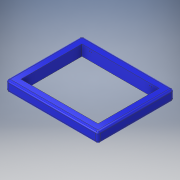
# Autodesk Inventor part: Wrap-Around Bumpers
Saved by Autodesk Inventor 2019 (Build 230136000, 136)
## iProperties
Created: 2018-11-17
Part Number: Wrap-Around Bumpers
Material: Generic
Document SubType Name: Modeling
Designer: maste
Density: 1 g/cm^3
Appearance: Default
Author: maste
Autodesk Inventor part; units mm, degrees
ref_plane "YZ Plane" through (0, 0, 0) normal (1, 0, 0) x (0, 1, 0)
ref_plane "XZ Plane" through (0, 0, 0) normal (0, 1, 0) x (-1, 0, 0)
ref_plane "XY Plane" through (0, 0, 0) normal (0, 0, 1) x (1, 0, 0)
sketch "Sketch1" plane through (0, 0, 0) normal (0, 0, 1) x (1, 0, 0)
  line L0 (0, 0) -> (914.4, 0)
  line L1 (914.4, 0) -> (914.4, 723.9)
  line L2 (914.4, 723.9) -> (0, 723.9)
  line L3 (0, 723.9) -> (0, 0)
  line L4 (-88.9, 812.8) -> (1003.3, 812.8)
  line L5 (1003.3, 812.8) -> (1003.3, -88.9)
  line L6 (1003.3, -88.9) -> (-88.9, -88.9)
  line L7 (-88.9, -88.9) -> (-88.9, 812.8)
  dimension "d0" = 914.4
  dimension "d1" = 723.9
  dimension "d2" = 88.9
  constraints: 16 end point, 4 parallel, 2 perpendicular, 1 horizontal, 3 other
  measures "d0" distance of L2.end L1.end
  measures "d1" distance of L1.end L0.end
  measures "d2" distance between parallel lines of L2 L4
extrude "Extrusion1" add sketch "Sketch1" along normal blind 127
sketch "Sketch2" plane through (1003.3, -88.9, 0) normal (1, 0, 0) x (0, 0, -1)
  line L0 (-101.3437, 557.5546) -> (-13.411, 557.5546) construction
  line L1 (-13.411, 557.5546) -> (-13.411, 343.9106) construction
  line L2 (-13.411, 343.9106) -> (-101.3437, 343.9106) construction
  line L3 (-101.3437, 343.9106) -> (-101.3437, 557.5546) construction
  line L4 (-99.1602, 555.4971) -> (-99.5233, 555.4971)
  line L5 (-99.5233, 555.4971) -> (-99.5233, 554.4498)
  line L6 (-99.5233, 554.4498) -> (-99.9161, 554.4498)
  line L7 (-99.9161, 554.4498) -> (-99.9161, 555.4971)
  line L8 (-99.9161, 555.4971) -> (-101.2622, 555.4971)
  line L9 (-101.2622, 555.4971) -> (-101.2622, 555.9269)
  line L10 (-101.2622, 555.9269) -> (-99.8988, 557.4978)
  line L11 (-99.8988, 557.4978) -> (-99.5233, 557.4978)
  line L12 (-99.5233, 557.4978) -> (-99.5233, 555.8256)
  line L13 (-99.5233, 555.8256) -> (-99.1602, 555.8256)
  line L14 (-99.1602, 555.8256) -> (-99.1602, 555.4971)
  line L15 (-99.9161, 555.8256) -> (-99.9161, 557.0161)
  line L16 (-99.9161, 557.0161) -> (-100.9411, 555.8256)
  line L17 (-100.9411, 555.8256) -> (-99.9161, 555.8256)
  line L18 (-96.873, 555.4971) -> (-97.2361, 555.4971)
  line L19 (-97.2361, 555.4971) -> (-97.2361, 554.4498)
  line L20 (-97.2361, 554.4498) -> (-97.6288, 554.4498)
  line L21 (-97.6288, 554.4498) -> (-97.6288, 555.4971)
  line L22 (-97.6288, 555.4971) -> (-98.975, 555.4971)
  line L23 (-98.975, 555.4971) -> (-98.975, 555.9269)
  line L24 (-98.975, 555.9269) -> (-97.6115, 557.4978)
  line L25 (-97.6115, 557.4978) -> (-97.2361, 557.4978)
  line L26 (-97.2361, 557.4978) -> (-97.2361, 555.8256)
  line L27 (-97.2361, 555.8256) -> (-96.873, 555.8256)
  line L28 (-96.873, 555.8256) -> (-96.873, 555.4971)
  line L29 (-97.6288, 555.8256) -> (-97.6288, 557.0161)
  line L30 (-97.6288, 557.0161) -> (-98.6539, 555.8256)
  line L31 (-98.6539, 555.8256) -> (-97.6288, 555.8256)
  spline S0 degree 2 poles (-94.6203, 555.4378) (-94.6203, 555.2032) (-94.776, 554.8055) (-94.9069, 554.6721) knots 0 0 0 1 2 2 2
  spline S1 degree 2 poles (-94.9069, 554.6721) (-95.0427, 554.5313) (-95.3836, 554.3856) (-95.5886, 554.3856) knots 0 0 0 1 2 2 2
  spline S2 degree 2 poles (-95.5886, 554.3856) (-95.7936, 554.3856) (-96.132, 554.5239) (-96.2604, 554.6622) knots 0 0 0 1 2 2 2
  spline S3 degree 2 poles (-96.2604, 554.6622) (-96.4185, 554.8277) (-96.5964, 555.3835) (-96.5964, 555.7885) knots 0 0 0 1 2 2 2
  spline S4 degree 2 poles (-96.5964, 555.7885) (-96.5964, 556.1862) (-96.4333, 556.826) (-96.2629, 557.0631) knots 0 0 0 1 2 2 2
  spline S5 degree 2 poles (-96.2629, 557.0631) (-96.0974, 557.2953) (-95.5738, 557.5546) (-95.2304, 557.5546) knots 0 0 0 1 2 2 2
  spline S6 degree 2 poles (-95.2304, 557.5546) (-95.1292, 557.5546) (-94.9513, 557.5348) (-94.8846, 557.5126) knots 0 0 0 1 2 2 2
  line L32 (-94.8846, 557.5126) -> (-94.8846, 557.1199)
  line L33 (-94.8846, 557.1199) -> (-94.9019, 557.1199)
  spline S7 degree 2 poles (-94.9019, 557.1199) (-94.9587, 557.1495) (-95.1662, 557.2014) (-95.2848, 557.2014) knots 0 0 0 1 2 2 2
  spline S8 degree 2 poles (-95.2848, 557.2014) (-95.6652, 557.2014) (-96.132, 556.6876) (-96.1765, 556.1838) knots 0 0 0 1 2 2 2
  spline S9 degree 2 poles (-96.1765, 556.1838) (-96.0307, 556.285) (-95.7244, 556.3962) (-95.5417, 556.3962) knots 0 0 0 1 2 2 2
  spline S10 degree 2 poles (-95.5417, 556.3962) (-95.3638, 556.3962) (-95.0971, 556.3245) (-94.9513, 556.2159) knots 0 0 0 1 2 2 2
  spline S11 degree 2 poles (-94.9513, 556.2159) (-94.7834, 556.0899) (-94.6203, 555.6996) (-94.6203, 555.4378) knots 0 0 0 1 2 2 2
  spline S12 degree 2 poles (-95.0353, 555.4205) (-95.0353, 555.6082) (-95.1341, 555.8626) (-95.2428, 555.9516) knots 0 0 0 1 2 2 2
  spline S13 degree 2 poles (-95.2428, 555.9516) (-95.3243, 556.0158) (-95.5268, 556.0578) (-95.633, 556.0578) knots 0 0 0 1 2 2 2
  spline S14 degree 2 poles (-95.633, 556.0578) (-95.7763, 556.0578) (-96.0455, 555.9713) (-96.1765, 555.8898) knots 0 0 0 1 2 2 2
  spline S15 degree 2 poles (-96.1765, 555.8898) (-96.1789, 555.8454) (-96.1839, 555.7614) (-96.1839, 555.6972) knots 0 0 0 1 2 2 2
  spline S16 degree 2 poles (-96.1839, 555.6972) (-96.1839, 555.381) (-96.0604, 554.9932) (-95.9665, 554.8919) knots 0 0 0 1 2 2 2
  spline S17 degree 2 poles (-95.9665, 554.8919) (-95.88, 554.7956) (-95.6923, 554.719) (-95.5861, 554.719) knots 0 0 0 1 2 2 2
  spline S18 degree 2 poles (-95.5861, 554.719) (-95.3391, 554.719) (-95.0353, 555.0698) (-95.0353, 555.4205) knots 0 0 0 1 2 2 2
  line L34 (-92.5332, 554.4498) -> (-94.0201, 554.4498)
  line L35 (-94.0201, 554.4498) -> (-94.0201, 554.761)
  line L36 (-94.0201, 554.761) -> (-93.4668, 554.761)
  line L37 (-93.4668, 554.761) -> (-93.4668, 556.8037)
  line L38 (-93.4668, 556.8037) -> (-94.0201, 556.8037)
  line L39 (-94.0201, 556.8037) -> (-94.0201, 557.0828)
  spline S19 degree 2 poles (-94.0201, 557.0828) (-93.7064, 557.0828) (-93.41, 557.2607) (-93.3903, 557.5077) knots 0 0 0 1 2 2 2
  line L40 (-93.3903, 557.5077) -> (-93.0741, 557.5077)
  line L41 (-93.0741, 557.5077) -> (-93.0741, 554.761)
  line L42 (-93.0741, 554.761) -> (-92.5332, 554.761)
  line L43 (-92.5332, 554.761) -> (-92.5332, 554.4498)
  point P0 (0, 88.9)
  constraints: 2 other
emboss "Emboss1" sketch "Sketch2" operation cut depth 2.54 direction (-1, 0, 0)
fillet "Fillet1" radius 25.4 12 edges at (457.2, 812.8, 0) (457.2, 812.8, 127) (1003.3, 812.8, 63.5) (1003.3, 361.95, 0) (1003.3, 361.95, 127) (1003.3, -88.9, 63.5) (457.2, -88.9, 127) (457.2, -88.9, 0) (-88.9, -88.9, 63.5) (-88.9, 361.95, 127) (-88.9, 361.95, 0) (-88.9, 812.8, 63.5)
sketch "Sketch3" plane through (0, 0, 0) normal (0, 1, 0) x (1, 0, 0)
  line L0 (0, 0) -> (914.4, 0) projected
  line L1 (0, 0) -> (0, -127) projected
  line L2 (0, 0) -> (0, -127)
  line L3 (0, -127) -> (0, -28.575)
  line L4 (0, -28.575) -> (1035.6793, -28.575)
  line L5 (0, -28.575) -> (101.6, -28.575)
  line L6 (101.6, -28.575) -> (101.6, -127)
  line L7 (914.4, -127) -> (0, -127) projected
  line L8 (101.6, -28.575) -> (88.9, -28.575)
  line L9 (101.6, -28.575) -> (114.3, -28.575)
  circle A0 centre (88.9, -28.575) radius 2.54
  circle A1 centre (114.3, -28.575) radius 2.54
  line L10 (457.2, 0) -> (457.2, -127)
  circle A2 centre (825.5, -28.575) radius 2.54
  circle A3 centre (800.1, -28.575) radius 2.54
  dimension "d8" = 98.425
  dimension "d9" = 101.6
  dimension "d10" = 12.7
  dimension "d11" = 12.7
  dimension "d12" = 5.08
  dimension "d13" = 5.08
  constraints: 16 end point, 5 point on line, 4 centre point, 2 coincident, 2 midpoint, 2 perpendicular, 2 symmetric about line, 1 vertical, 2 other
  measures "d8" distance of L1.end L3.end
  measures "d9" distance of L3.end L5.end
  measures "d10" distance of L5.end L8.end
  measures "d11" distance of L5.end L9.end
  measures "d12" diameter of A0
  measures "d13" diameter of A1
extrude "Extrusion2" cut sketch "Sketch3" against normal blind 2.54 contours A0 L4 | L4 A0 | A1 L4 | L4 A1 | A3 L4 | L4 A3 | A2 L4 | L4 A2
body "Solid1"
